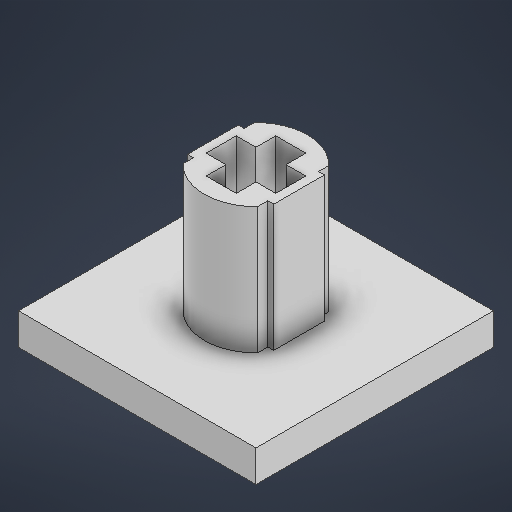
# Autodesk Inventor part: button_3d
Saved by Autodesk Inventor 2026 (Build 300175000, 175)
## iProperties
Created: 2025-05-11
Part Number: button_3d
Material: 일반
Document SubType Name: Modeling
Designer: encle
Density: 1 g/cm^3
Appearance: 기본값
Author: encle
Autodesk Inventor part; units mm, degrees
ref_plane "YZ Plane" through (0, 0, 0) normal (1, 0, 0) x (0, 1, 0)
ref_plane "XZ Plane" through (0, 0, 0) normal (0, 1, 0) x (-1, 0, 0)
ref_plane "XY Plane" through (0, 0, 0) normal (0, 0, 1) x (1, 0, 0)
sketch "스케치6" plane through (0, 0, 0) normal (0, 1, 0) x (-1, 0, 0)
  line L0 (-7.5, 7.5) -> (7.5, 7.5)
  line L1 (7.5, 7.5) -> (7.5, -7.5)
  line L2 (7.5, -7.5) -> (-7.5, -7.5)
  line L3 (-7.5, -7.5) -> (-7.5, 7.5)
  line L4 (-7.5, 7.5) -> (7.5, -7.5) construction
  line L5 (7.5, 7.5) -> (-7.5, -7.5) construction
  point P0 (0, 0)
  dimension "d20" = 15
  dimension "d21" = 15
  constraints: 12 end point, 2 midpoint, 2 parallel, 1 horizontal, 1 perpendicular
  measures "d20" distance of L1.end L2.end
  measures "d21" distance of L0.end L1.end
extrude "돌출4" add sketch "스케치6" along normal blind 2
sketch "스케치7" plane through (0, 2, 0) normal (0, 1, 0) x (1, 0, 0)
  line L0 (2.2, -0.95) -> (2.2, 0.95)
  line L1 (-2.2, 0.95) -> (-2.2, -0.95)
  line L2 (-0.95, -2.2) -> (0.95, -2.2)
  line L3 (0.95, 2.2) -> (-0.95, 2.2)
  line L4 (2.2, 0.95) -> (0.95, 0.95)
  line L5 (-0.95, 0.95) -> (-2.2, 0.95)
  line L6 (-0.95, 2.2) -> (-0.95, 0.95)
  line L7 (-0.95, -0.95) -> (-0.95, -2.2)
  line L8 (-2.2, -0.95) -> (-0.95, -0.95)
  line L9 (0.95, -0.95) -> (2.2, -0.95)
  line L10 (0.95, -2.2) -> (0.95, -0.95)
  line L11 (0.95, 0.95) -> (0.95, 2.2)
  circle A0 centre (0, 0) radius 3.25
  line L12 (-2.35, -2.245) -> (-2.35, 2.245)
  line L13 (2.35, -2.245) -> (2.35, 2.245)
  line L14 (2.35, 1.6) -> (2.725, 1.6)
  line L15 (2.725, 1.6) -> (2.725, -1.6)
  line L16 (2.725, -1.6) -> (2.35, -1.6)
  line L17 (2.35, -1.6) -> (2.35, 1.6)
  line L18 (-2.35, 1.6) -> (-2.725, 1.6)
  line L19 (-2.725, 1.6) -> (-2.725, -1.6)
  line L20 (-2.725, -1.6) -> (-2.35, -1.6)
  line L21 (-2.35, -1.6) -> (-2.35, 1.6)
  point P0 (2.5375, 1.6)
  point P1 (2.5375, -1.6)
  dimension "d24" = 0.95
  dimension "d25" = 1.9
  dimension "d26" = 0.95
  dimension "d27" = 1.9
  dimension "d28" = 4.4
  dimension "d29" = 4.4
  dimension "d30" = 6.5
  dimension "d31" = 4.7
  dimension "d32" = 1.6
  dimension "d33" = 3.2
  dimension "d34" = 0.375
  constraints: 44 end point, 14 parallel, 6 collinear, 6 perpendicular, 5 horizontal, 4 equal length, 4 point on circle, 2 midpoint, 2 point on line, 2 vertical, 1 centre point, 1 coincident
  measures "d24" distance from line of point (0, 0) L5
  measures "d25" distance of L1.start L1.end
  measures "d26" distance from line of L6 point (0, 0)
  measures "d27" distance between parallel lines of L11 L6
  measures "d28" distance between parallel lines of L3 L2
  measures "d29" distance between parallel lines of L1 L0
  measures "d30" diameter of A0
  measures "d31" distance between parallel lines of L13 L12
  measures "d32" vertical distance of A0.centre point (2.538, 1.6)
  measures "d33" distance of point (2.538, -1.6) point (2.538, 1.6)
  measures "d34" distance of L14.start L14.end
extrude "돌출5" add sketch "스케치7" along normal blind 8 contours L13 A0 L12 | L14 L15 L16 L13 | L12 L20 L19 L18
equation "\"d24\" = 0.5 * d25"
equation "\"d26\" = 0.5 * d27"
equation "\"d32\" = 0.5 * d33"
